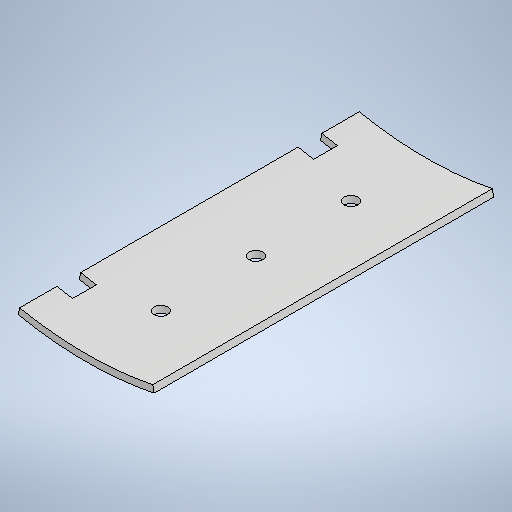
# Autodesk Inventor part: 214,2
Saved by Autodesk Inventor 2025 (Build 290162010, 162A)
## iProperties
Created: 2024-06-09
Part Number: 214,2
Material: Generic
Document SubType Name: Modeling
Designer: Fabri
Density: 1 g/cm^3
Appearance: Default
Author: Fabri
Autodesk Inventor part; units mm, degrees
ref_plane "YZ Plane" through (0, 0, 0) normal (1, 0, 0) x (0, 1, 0)
ref_plane "XZ Plane" through (0, 0, 0) normal (0, 1, 0) x (-1, 0, 0)
sketch "Sketch1" plane through (0, 0, 0) normal (0, 1, 0) x (-1, 0, 0)
  arc A0 (-19.604, -97.0396) -> (19.604, -97.0396) centre (0, 0) ccw
  line L0 (19.604, -97.0396) -> (20, -99)
  line L1 (-19.604, -97.0396) -> (-20, -99)
  arc A1 (-20, -99) -> (20, -99) centre (0, 0) ccw
  line L2 (0, 0) -> (0, 18.8083) construction
  point P0 (0, -99)
  point P1 (0, -101)
  dimension "d0" = 2
  dimension "d1" = 101
  dimension "d2" = 40
  dimension "d3" = 99
  constraints: 6 end point, 6 point on circle, 4 coincident, 2 centre point, 2 vertical alignment, 1 vertical, 1 other
  measures "d0" distance of L0.start L0.end
  measures "d1" radius of A1
  measures "d2" distance of L1.end L0.end
  measures "d3" radius of A0
extrude "Extrusion1" add sketch "Sketch1" along normal blind 100
ref_plane "Work Plane1" through (0, 0, -101) normal (0, 0, -1) x (-1, 0, 0)
sketch "Sketch2" plane through (0, 0, -101) normal (0, 0, -1) x (-1, 0, 0)
  line L0 (-20, 0) -> (20, 0) projected
  line L1 (20, 0) -> (20, 100) projected
  line L2 (-20, 100) -> (20, 100) projected
  line L3 (-20, 0) -> (-20, 100) projected
  point P0 (0, 0)
  point P1 (0, 22)
  point P2 (0, 22)
  point P3 (0, 50)
  point P4 (0, 78)
  point P5 (0, 100)
  dimension "d7" = 22
  dimension "d8" = 22
  dimension "d9" = 28
  dimension "d10" = 28
  constraints: 4 vertical alignment, 1 midpoint
  measures "d7" distance from line of point (0, 78) L2
  measures "d8" distance from line of L0 point (0, 22)
  measures "d9" distance of point (0, 50) point (0, 78)
  measures "d10" distance of point (0, 22) point (0, 50)
hole "Hole1" at (0, 22, -101) at (0, 50, -101) at (0, 78, -101) direction (0, 0, 1) diameter 4 end through all
sketch "Sketch3" plane through (0, 0, -101) normal (0, 0, -1) x (-1, 0, 0)
  line L0 (20, 0) -> (20, 100) projected
  line L1 (20, 100) -> (-20, 100) projected
  line L2 (20, 0) -> (-20, 0) projected
  line L3 (20, 89) -> (15, 89)
  line L4 (15, 89) -> (15, 82)
  line L5 (15, 82) -> (20, 82)
  line L6 (20, 18) -> (15, 18)
  line L7 (15, 18) -> (15, 11)
  line L8 (15, 11) -> (20, 11)
  point P0 (0, 0)
  point P1 (0, 52)
  point P2 (0, 48)
  dimension "d18" = 7
  dimension "d19" = 5
  dimension "d20" = 11
  dimension "d21" = 5
  dimension "d22" = 11
  dimension "d23" = 7
  constraints: 12 end point, 4 perpendicular, 4 point on line, 2 horizontal, 2 vertical alignment
  measures "d18" distance of L3.end L4.end
  measures "d19" distance between parallel lines of L0 L4
  measures "d20" distance between parallel lines of L3 L1
  measures "d21" distance between parallel lines of L7 L0
  measures "d22" distance between parallel lines of L2 L8
  measures "d23" distance between parallel lines of L8 L6
extrude "Extrusion2" cut sketch "Sketch3" against normal up to surface
equation "\"d8\" = d7"
equation "\"d10\" = d9"
body "Solid1"
